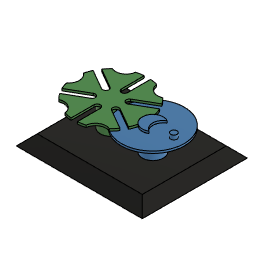
homework nr 4.2 good (Autodesk Fusion 360 design; units mm, degrees)
Autodesk Fusion 360 part; units mm, degrees
note: some values were not read from the file. Set by a fixed rule: which sketch regions a step uses.
sketch "schita baza" plane through (0, 0, 0) normal (0, 0, 1) x (1, 0, 0) in component "baza"
  line L0 (300, 250) -> (-300, 250)
  line L1 (-300, 250) -> (-300, -250)
  line L2 (-300, -250) -> (300, -250)
  line L3 (300, -250) -> (300, 250)
  line L4 (300, 250) -> (-300, -250) construction
  line L5 (-300, 250) -> (300, -250) construction
  dimension "d1" = 600
  dimension "d2" = 500
  constraint horizontal L0
  constraint perpendicular L0 L1
  constraint parallel L0 L2
  constraint parallel L1 L3
  constraint coincident L4 origin
  constraint coincident L5 origin
  measures "d1" distance of L1.end L2.end
  measures "d2" distance of L0.end L1.end
extrude "Extrude1" add sketch "schita baza" along normal blind 50 makes body 1 in component "baza"
chamfer "Chamfer1" distance 50 angle 45 1 faces at (-100, 83.3333, 50) on bodies 1 in component "baza"
sketch "piciot rotita" plane through (0, 0, 50) normal (0, 0, 1) x (-1, 0, 0) in component "picior rotita"
  line L0 (250, -200) -> (250, 200)
  line L1 (250, 200) -> (-250, 200)
  line L2 (-250, 200) -> (-250, -200)
  line L3 (-250, -200) -> (250, -200)
  circle A0 centre (-100, 0) radius 50
  circle A1 centre (-100, 0) radius 50.2
  dimension "d6" = 100
  dimension "d70" = 0.2
  measures "d6" distance of origin A0.centre
extrude "Extrude1'" add sketch "piciot rotita" along normal blind 100 and the other way blind 20 separate body contours A0 makes body 2 in component "picior rotita"
sketch "corp rotita" plane through (0, 0, 150) normal (0, 0, 1) x (-1, 0, 0) in component "rotita"
  circle A0 centre (-100, 0) radius 50
  circle A1 centre (-100, 0) radius 150
  dimension "d9" = 300
  constraint concentric A0 A1
  measures "d9" diameter of A1
extrude "Extrude1''" add sketch "corp rotita" along normal blind 10 separate body contours A0 | A1 makes body 3 in component "rotita"
sketch "ax" plane through (0, 0, 160) normal (0, 0, 1) x (-1, 0, 0) in component "rotita"
  circle A0 centre (-100, 0) radius 150
  circle A1 centre (-100, 0) radius 10
  circle A2 centre (-100, 0) radius 10.3
  dimension "d12" = 0.3
  constraint concentric A0 A1
extrude "Extrude2" add sketch "ax" against normal blind 160 contours A1 bodies 3 in component "rotita"
extrude "Extrude2'" cut sketch "ax" against normal blind 110 contours A1 | A2 bodies 2 in component "picior rotita"
extrude "Extrude2''" cut sketch "ax" against normal blind 160 contours A1 | A2 bodies 1 in component "baza"
sketch "MODELE " plane through (0, 0, 160) normal (0, 0, 1) x (-1, 0, 0) in component "rotita"
  circle A0 centre (-199.9989, -0.3314) radius 15
  arc A1 (-125, -43.3013) -> (-125, 43.3013) centre (-150, 0) ccw
  arc A2 (-197.8473, 14.5134) -> (-197.6506, -15.1465) centre (-150, 0) ccw
  arc A3 (-125, -43.3013) -> (-125, 43.3013) centre (-100, 0) ccw
  dimension "d19" = 100
  dimension "d20" = 100
  dimension "d21" = 30
  constraint coincident A1.centre A3
  constraint coincident A0.centre A1
  constraint coincident A0 A2.end
  constraint coincident A0 A2.start
  constraint concentric A1 A2
  measures "d19" diameter of A3
  measures "d20" diameter of A1
  measures "d21" diameter of A0
extrude "Extrude3" add sketch "MODELE " along normal blind 10 contours A1 A3 bodies 3 in component "rotita"
extrude "Extrude4" add sketch "MODELE " along normal blind 20 contours A0 A2 | A0 A2 bodies 3 in component "rotita"
sketch "BAZA ROATA" plane through (0, 0, 50) normal (0, 0, 1) x (-1, 0, 0) in component "BAZA ROATA FLOARE"
  circle A0 centre (-100, 0) radius 10.3
  line L0 (250, -200) -> (250, 200)
  line L1 (250, 200) -> (-250, 200)
  line L2 (-250, 200) -> (-250, -200)
  line L3 (-250, -200) -> (250, -200)
  circle A1 centre (100, 0) radius 50
  circle A2 centre (100, 0) radius 50.2
  dimension "d26" = 100
  dimension "d65" = 0.2
  measures "d26" diameter of A1
extrude "Extrude1'''" add sketch "BAZA ROATA" along normal blind 110 and the other way blind 20 separate body contours A1 makes body 4 in component "BAZA ROATA FLOARE"
sketch "MODEL FLOARE" plane through (0, 0, 160) normal (0, 0, 1) x (-1, 0, 0) in component "ROATA FLOARE"
  circle A0 centre (-199.9989, -0.3314) radius 15
  arc A1 (-125, -43.3013) -> (-125, 43.3013) centre (-150, 0) ccw
  arc A2 (-125, -43.3013) -> (-125, 43.3013) centre (-100, 0) ccw
  circle A3 centre (-100, 0) radius 150
  line L0 (-250, -0.0001) -> (-214.9952, -0.0001)
  line L1 (-100, 0) -> (-100, -150) construction
  line L2 (-100, 0) -> (-100, 150) construction
  circle A4 centre (-100, 0) radius 114.9995 construction
  circle A5 centre (-100, 0) radius 84.9995 construction
  circle A6 centre (100, 0) radius 50
  line L3 (36.2083, -19.5096) -> (-58.4967, -74.1876)
  line L4 (51.2083, -45.4904) -> (-43.4967, -100.1684)
  line L5 (85, -65) -> (85, -174.356)
  line L6 (115, -65) -> (115, -174.356)
  line L7 (148.7917, -45.4904) -> (243.4967, -100.1684)
  line L8 (163.7917, -19.5096) -> (258.4967, -74.1876)
  line L9 (163.7917, 19.5096) -> (258.4967, 74.1876)
  line L10 (148.7917, 45.4904) -> (243.4967, 100.1684)
  line L11 (115, 65) -> (115, 174.356)
  line L12 (85, 65) -> (85, 174.356)
  line L13 (51.2083, 45.4904) -> (-43.4967, 100.1684)
  line L14 (36.2083, 19.5096) -> (-58.4967, 74.1876)
  arc A7 (115, -65) -> (85, -65) centre (100, -65) ccw
  arc A8 (42.3026, -47.434) -> (36.2083, -19.5096) centre (43.7083, -32.5) ccw
  arc A9 (36.2083, 19.5096) -> (42.3026, 47.434) centre (43.7083, 32.5) ccw
  arc A10 (85, 65) -> (115, 65) centre (100, 65) ccw
  arc A11 (148.7917, 45.4904) -> (163.7917, 19.5096) centre (156.2917, 32.5) ccw
  arc A12 (163.7917, -19.5096) -> (148.7917, -45.4904) centre (156.2917, -32.5) ccw
  arc A13 (-70.3125, -40.2325) -> (-70.3125, 40.2325) centre (-100, 0) ccw
  arc A14 (-25, 129.9038) -> (49.6861, 167.6112) centre (0, 173.2051) ccw
  arc A15 (150.3139, 167.6112) -> (219.9986, 127.3787) centre (200, 173.2051) ccw
  arc A16 (270.3125, 40.2325) -> (270.3125, -40.2325) centre (300, 0) ccw
  arc A17 (219.9986, -127.3787) -> (150.3139, -167.6112) centre (200, -173.2051) ccw
  arc A18 (49.6861, -167.6112) -> (-25, -129.9038) centre (0, -173.2051) ccw
  arc A19 (258.4967, -74.1876) -> (270.3125, -40.2325) centre (100, 0) ccw
  arc A20 (270.3125, 40.2325) -> (258.4967, 74.1876) centre (100, 0) ccw
  arc A21 (115, -174.356) -> (150.3139, -167.6112) centre (100, 0) ccw
  arc A22 (219.9986, -127.3787) -> (243.4967, -100.1684) centre (100, 0) ccw
  arc A23 (-43.5003, -100.1632) -> (-19.9986, -127.3787) centre (100, 0) ccw
  arc A24 (49.6861, -167.6112) -> (85, -174.356) centre (100, 0) ccw
  arc A25 (-58.4967, 74.1876) -> (-70.3125, 40.2325) centre (100, 0) ccw
  arc A26 (-70.3125, -40.2325) -> (-58.4967, -74.1876) centre (100, 0) ccw
  arc A27 (85, 174.356) -> (49.6861, 167.6112) centre (100, 0) ccw
  arc A28 (-19.9986, 127.3787) -> (-43.5003, 100.1632) centre (100, 0) ccw
  arc A29 (243.4967, 100.1684) -> (219.9986, 127.3787) centre (100, 0) ccw
  arc A30 (150.3139, 167.6112) -> (115, 174.356) centre (100, 0) ccw
  dimension "d29" = 35.0048
  dimension "d32" = 100
  dimension "d34" = 30
  constraint coincident A3 L0.start
  constraint coincident A0 L0.end
  constraint horizontal L0
  constraint coincident A2.centre A3.centre
  constraint coincident A3 L1.end
  constraint tangent A1 L1
  constraint vertical L1
  constraint coincident A3 L2.end
  constraint tangent A1 L2
  constraint parallel L1 L2
  constraint tangent A0 A4
  constraint tangent A0 A5
  constraint concentric A6 A21
  constraint tangent L3 A8
  constraint coincident L4.start A8
  constraint coincident L4.end A21
  constraint tangent L4 A8
  constraint parallel L3 L4
  constraint coincident A3 A8.start
  constraint coincident A3 A9.end
  constraint coincident A13.end A21
  constraint coincident A13.start A21
  constraint coincident A14.end A21
  constraint coincident A3 A14.start
  constraint coincident A15.end A21
  constraint coincident A15.start A21
  constraint coincident A16.end A21
  constraint coincident A16.start A21
  constraint coincident A17.start A21
  constraint coincident A3 A18.end
  constraint coincident A18.start A21
  constraint coincident A4 A23.start
  constraint concentric A21 A23
  constraint coincident A4 A28.end
  constraint concentric A21 A25
  constraint concentric A21 A27
  constraint concentric A21 A29
  constraint concentric A19 A21
  constraint concentric A19 A20
  constraint concentric A21 A22
  constraint coincident A18 A23.end
  constraint concentric A23 A24
  constraint concentric A25 A26
  constraint coincident A14 A28.start
  constraint concentric A27 A28
  constraint concentric A29 A30
  measures "d29" distance of L0.start L0.end
  measures "d32" diameter of A6
  measures "d34" diameter of A8
extrude "Extrude1''''" add sketch "MODEL FLOARE" along normal blind 10 separate body contours A2 A3 L3 L14 A8 A9 A13 A25 A26 | A3 A6 A8 | A3 A6 A9 | A6 | A3 A6 L4 L5 A7 A8 A18 A23 A24 | A3 A6 L12 L13 A9 A10 A14 A27 A28 | A3 L4 A23 | A6 L6 L7 A7 A12 A17 A21 A22 | A3 L13 A28 | A6 L10 L11 A10 A11 A15 A29 A30 | A6 L8 L9 A11 A12 A16 A19 A20 makes body 5 in component "ROATA FLOARE"
sketch "AX FLOARE" plane through (0, 0, 170) normal (0, 0, 1) x (-1, 0, 0) in component "ROATA FLOARE"
  line L0 (148.7917, 45.4904) -> (243.4967, 100.1684)
  arc A0 (243.4967, 100.1684) -> (219.9986, 127.3787) centre (100, 0) ccw
  arc A1 (150.3139, 167.6112) -> (219.9986, 127.3787) centre (200, 173.2051) ccw
  arc A2 (150.3139, 167.6112) -> (115, 174.356) centre (100, 0) ccw
  line L1 (115, 174.356) -> (115, 65)
  arc A3 (85, 65) -> (115, 65) centre (100, 65) ccw
  line L2 (85, 65) -> (85, 174.356)
  arc A4 (85, 174.356) -> (49.6861, 167.6112) centre (100, 0) ccw
  arc A5 (-19.9986, 127.3787) -> (49.6861, 167.6112) centre (0, 173.2051) ccw
  arc A6 (-19.9986, 127.3787) -> (-43.4967, 100.1684) centre (100, 0) ccw
  line L3 (-43.4967, 100.1684) -> (51.2083, 45.4904)
  arc A7 (36.2083, 19.5096) -> (51.2083, 45.4904) centre (43.7083, 32.5) ccw
  line L4 (36.2083, 19.5096) -> (-58.4967, 74.1876)
  arc A8 (-58.4967, 74.1876) -> (-70.3125, 40.2325) centre (100, 0) ccw
  arc A9 (-70.3125, -40.2325) -> (-70.3125, 40.2325) centre (-100, 0) ccw
  arc A10 (-70.3125, -40.2325) -> (-58.4967, -74.1876) centre (100, 0) ccw
  line L5 (-58.4967, -74.1876) -> (36.2083, -19.5096)
  arc A11 (51.2083, -45.4904) -> (36.2083, -19.5096) centre (43.7083, -32.5) ccw
  line L6 (51.2083, -45.4904) -> (-43.4967, -100.1684)
  arc A12 (-43.4967, -100.1684) -> (-19.9986, -127.3787) centre (100, 0) ccw
  arc A13 (49.6861, -167.6112) -> (-19.9986, -127.3787) centre (0, -173.2051) ccw
  arc A14 (49.6861, -167.6112) -> (85, -174.356) centre (100, 0) ccw
  line L7 (85, -174.356) -> (85, -65)
  arc A15 (115, -65) -> (85, -65) centre (100, -65) ccw
  line L8 (115, -65) -> (115, -174.356)
  arc A16 (115, -174.356) -> (150.3139, -167.6112) centre (100, 0) ccw
  arc A17 (219.9986, -127.3787) -> (150.3139, -167.6112) centre (200, -173.2051) ccw
  arc A18 (219.9986, -127.3787) -> (243.4967, -100.1684) centre (100, 0) ccw
  line L9 (243.4967, -100.1684) -> (148.7917, -45.4904)
  arc A19 (163.7917, -19.5096) -> (148.7917, -45.4904) centre (156.2917, -32.5) ccw
  line L10 (163.7917, -19.5096) -> (258.4967, -74.1876)
  arc A20 (258.4967, -74.1876) -> (270.3125, -40.2325) centre (100, 0) ccw
  arc A21 (270.3125, 40.2325) -> (270.3125, -40.2325) centre (300, 0) ccw
  arc A22 (270.3125, 40.2325) -> (258.4967, 74.1876) centre (100, 0) ccw
  line L11 (258.4967, 74.1876) -> (163.7917, 19.5096)
  arc A23 (148.7917, 45.4904) -> (163.7917, 19.5096) centre (156.2917, 32.5) ccw
  circle A24 centre (100, 0) radius 10
  circle A25 centre (100, 0) radius 10.3
  dimension "d41" = 20
  dimension "d42" = 0.3
  constraint concentric A0 A24
  measures "d41" diameter of A24
extrude "Extrude2'''" add sketch "AX FLOARE" against normal blind 170 contours A24 bodies 5 in component "ROATA FLOARE"
extrude "Extrude2''''" cut sketch "AX FLOARE" against normal blind 120 contours A24 | A25 bodies 4 in component "BAZA ROATA FLOARE"
extrude "Extrude3'" cut sketch "AX FLOARE" against normal blind 170 contours A24 | A25 bodies 1 in component "baza"
extrude "Extrude4'" cut sketch "BAZA ROATA" against normal blind 20 contours A1 | A2 bodies 1 in component "baza"
extrude "Extrude5" cut sketch "piciot rotita" against normal blind 20 contours A0 | A1 bodies 1 in component "baza"
component "baza" placed x (1, 0, 0) y (0, 1, 0) z (0, 0, 1) at (0, 0, 0)
component "picior rotita" placed x (1, 0, 0) y (0, 1, 0) z (0, 0, 1) at (0, 0, 0)
component "rotita" placed x (1, 0, 0) y (0, 1, 0) z (0, 0, 1) at (0, 0, 0)
component "ROATA FLOARE" placed x (1, 0, 0) y (0, 1, 0) z (0, 0, 1) at (0, 0, 0)
component "BAZA ROATA FLOARE" placed x (1, 0, 0) y (0, 1, 0) z (0, 0, 1) at (0, 0, 0)
named bodies: "baza", "picior rotita", "rotita", "BAZA ROATA FLOARE", "FLOARE"
